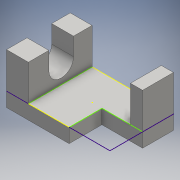
# Autodesk Inventor part: 240510_3Dsketch03
Saved by Autodesk Inventor 2016 (Build 200138000, 138)
## iProperties
Created: 2024-05-10
Part Number: 240510_3Dsketch03
Material: 일반
Document SubType Name: Modeling
Designer: pc
Density: 1 g/cm^3
Appearance: 기본값
Author: pc
Autodesk Inventor part; units mm, degrees
ref_plane "YZ Plane" through (0, 0, 0) normal (1, 0, 0) x (0, 1, 0)
ref_plane "XZ Plane" through (0, 0, 0) normal (0, 1, 0) x (-1, 0, 0)
ref_plane "XY Plane" through (0, 0, 0) normal (0, 0, 1) x (1, 0, 0)
sketch "스케치1" plane through (0, 0, 0) normal (0, 0, 1) x (1, 0, 0)
  line L0 (-36.8843, 21.5147) -> (35.1087, 21.5147)
  line L1 (35.1087, 21.5147) -> (35.1087, -22.8868)
  line L2 (35.1087, -22.8868) -> (-36.8843, -22.8868)
  line L3 (-36.8843, -22.8868) -> (-36.8843, 21.5147)
  point P0 (0, 0)
  constraints: 8 end point, 2 parallel, 1 horizontal, 1 perpendicular
extrude "돌출1" add sketch "스케치1" along normal blind 10
sketch "스케치2" plane through (0, 0, 10) normal (0, 0, 1) x (1, 0, 0)
  line L0 (-36.8843, -22.8868) -> (35.1087, -22.8868) projected
  line L1 (35.1087, -22.8868) -> (35.1087, 21.5147) projected
  line L2 (6.7199, -22.8868) -> (35.1087, -22.8868)
  line L3 (35.1087, -22.8868) -> (35.1087, 0)
  line L4 (35.1087, 0) -> (6.7199, 0)
  line L5 (6.7199, 0) -> (6.7199, -22.8868)
  line L6 (26.6326, 0) -> (35.1087, 0)
  line L7 (35.1087, 0) -> (35.1087, 21.5147)
  line L8 (35.1087, 21.5147) -> (26.6326, 21.5147)
  line L9 (26.6326, 21.5147) -> (26.6326, 0)
  line L10 (35.1087, 21.5147) -> (-36.8843, 21.5147) projected
  line L11 (-36.8843, -22.8868) -> (-21.6685, -22.8868)
  line L12 (-21.6685, -22.8868) -> (-21.6685, 21.5147)
  line L13 (-21.6685, 21.5147) -> (-36.8843, 21.5147)
  line L14 (-36.8843, 21.5147) -> (-36.8843, -22.8868)
  point P0 (0, 0)
  constraints: 24 end point, 6 parallel, 4 point on line, 3 horizontal, 3 perpendicular
extrude "돌출2" cut sketch "스케치2" against normal blind 10 contours L5 L4 L1 L0
extrude "돌출3" add sketch "스케치2" along normal blind 25 contours L8 L1 L4 L9
extrude "돌출4" add sketch "스케치2" along normal blind 25 contours L14 L10 L12 L0
sketch "스케치3" plane through (-36.8843, -22.8868, 0) normal (-1, 0, 0) x (0, 0, 1)
  arc A0 (22.6138, 31.4883) -> (22.6138, 14.2853) centre (22.6138, 22.8868) ccw
  line L0 (22.6138, 31.4883) -> (34.7327, 31.4883)
  line L1 (22.6138, 14.2853) -> (34.7327, 14.2853)
  point P0 (0, 22.8868)
  constraints: 4 end point, 2 horizontal, 2 point on circle, 1 centre point
extrude "돌출5" cut sketch "스케치3" against normal blind 25 fills toward (28.6733, 31.4383) open curves L0 A0 L1
